Autodesk Fusion 360 part; units mm, degrees
note: some values were not read from the file. Set by a fixed rule: which sketch regions a step uses.
(part 3 of 3)
sketch "Sketch8" plane through (0, 0, 0) normal (0, 0, -1) x (1, 0, 0)
  line L0 (182.6113, -19.0647) -> (183.6113, -17.3326)
  line L1 (183.6113, -17.3326) -> (182.6113, -15.6006)
  line L2 (182.6113, -15.6006) -> (183.6113, -13.8685)
  line L3 (183.6113, -13.8685) -> (182.6113, -12.1365)
  line L4 (182.6113, -12.1365) -> (183.6113, -10.4044)
  line L5 (183.6113, -10.4044) -> (182.6113, -8.6724)
  line L6 (182.6113, -8.6724) -> (183.6113, -6.9403)
  line L7 (183.6113, -6.9403) -> (182.6113, -5.2083)
  line L8 (182.6113, -5.2083) -> (183.6113, -3.4762)
  line L9 (183.6113, -3.4762) -> (182.6113, -1.7442)
  line L10 (182.6113, -1.7442) -> (183.6113, -0.0121)
  line L11 (183.6113, -0.0121) -> (183.6113, 1.6298)
  line L12 (183.6113, 1.6298) -> (176, 1.6298)
  line L13 (176, 1.6298) -> (176, -7.1298)
  arc A0 (173.5, -11.4599) -> (176, -7.1298) centre (171, -7.1298) ccw
  line L14 (173.5, -11.4599) -> (170.6456, -13.1079)
  arc A1 (170.6456, -13.1079) -> (170.1456, -13.9739) centre (171.1456, -13.9739) ccw
  line L15 (170.1456, -13.9739) -> (170.1456, -15.2165)
  arc A2 (169.9665, -15.4154) -> (170.1456, -15.2165) centre (169.9456, -15.2165) ccw
  line L16 (169.9665, -15.4154) -> (167.3665, -15.6887)
  arc A3 (167.1456, -15.4898) -> (167.3665, -15.6887) centre (167.3456, -15.4898) ccw
  line L17 (167.1456, -15.4898) -> (167.1456, -15.4119)
  line L18 (167.1456, -15.4119) -> (151.6323, -17.0424)
  line L19 (151.6323, -17.0424) -> (151.6323, -17.1623)
  arc A4 (151.4532, -17.3612) -> (151.6323, -17.1623) centre (151.4323, -17.1623) ccw
  line L20 (151.4532, -17.3612) -> (148.8532, -17.6345)
  arc A5 (148.6323, -17.4356) -> (148.8532, -17.6345) centre (148.8323, -17.4356) ccw
  line L21 (148.6323, -17.4356) -> (148.6323, -15.55)
  arc A6 (148.6323, -15.55) -> (148.3823, -15.3) centre (148.3823, -15.55) ccw
  line L22 (148.3823, -15.3) -> (148.1323, -15.3)
  spline S0 degree 5 poles (148.1323, -15.3) (148.4158, -14.6516) (148.9812, -13.354) (149.8244, -11.4057) (150.9388, -8.8038) (152.3141, -5.5444) (153.6703, -2.2771) (155.0058, 0.9987) (156.3196, 4.2834) (157.6127, 7.5765) (158.8598, 10.8079) (159.8388, 13.3845) (160.5594, 15.3025) (161.0282, 16.559) (161.2489, 17.1526) knots 0 0 0 0 0 0 0.1 0.2 0.3 0.4 0.5 0.6 0.7 0.8 0.9 0.989467 0.989467 0.989467 0.989467 0.989467 0.989467
  arc A7 (161.7176, 17.4784) -> (161.2489, 17.1526) centre (161.7176, 16.9784) ccw
  line L23 (161.7176, 17.4784) -> (162.4215, 17.4784)
  arc A8 (162.9139, 17.0652) -> (162.4215, 17.4784) centre (162.4215, 16.9784) ccw
  line L24 (162.9139, 17.0652) -> (165.3864, 3.043)
  arc A9 (165.3864, 3.043) -> (165.8788, 2.6298) centre (165.8788, 3.1298) ccw
  line L25 (165.8788, 2.6298) -> (184.9592, 2.6298)
  arc A10 (185.4592, 2.1298) -> (184.9592, 2.6298) centre (184.9592, 2.1298) ccw
  line L26 (185.4592, 2.1298) -> (185.4592, -0.0467)
  line L27 (185.4592, -0.0467) -> (186.4393, -1.7442)
  line L28 (186.4393, -1.7442) -> (185.4393, -3.4762)
  line L29 (185.4393, -3.4762) -> (186.4393, -5.2083)
  line L30 (186.4393, -5.2083) -> (185.4393, -6.9403)
  line L31 (185.4393, -6.9403) -> (186.4393, -8.6724)
  line L32 (186.4393, -8.6724) -> (185.4393, -10.4044)
  line L33 (185.4393, -10.4044) -> (186.4393, -12.1365)
  line L34 (186.4393, -12.1365) -> (185.4393, -13.8685)
  line L35 (185.4393, -13.8685) -> (186.4393, -15.6006)
  line L36 (186.4393, -15.6006) -> (185.4393, -17.3326)
  line L37 (185.4393, -17.3326) -> (186.4393, -19.0647)
  line L38 (186.4393, -19.0647) -> (185.4393, -20.7967)
  line L39 (185.4393, -20.7967) -> (189.0932, -28.2505)
  arc A11 (189.0932, -28.2505) -> (190.889, -29.3702) centre (190.889, -27.3702) ccw
  line L40 (190.889, -29.3702) -> (197.156, -29.3702)
  arc A12 (197.156, -29.3702) -> (202.156, -24.3702) centre (197.156, -24.3702) ccw
  line L41 (202.156, -24.3702) -> (202.156, 8.9998)
  line L42 (202.156, 8.9998) -> (186.578, 8.932)
  arc A13 (186.578, 8.932) -> (186.0802, 8.4298) centre (186.5802, 8.432) ccw
  line L43 (186.0802, 8.4298) -> (186.0859, 7.132)
  arc A14 (185.5859, 6.6298) -> (186.0859, 7.132) centre (185.5859, 7.1298) ccw
  line L44 (185.5859, 6.6298) -> (178.088, 6.6298)
  arc A15 (177.588, 7.1298) -> (178.088, 6.6298) centre (178.088, 7.1298) ccw
  line L45 (177.588, 7.1298) -> (177.588, 23.1298)
  arc A16 (178.088, 23.6298) -> (177.588, 23.1298) centre (178.088, 23.1298) ccw
  line L46 (178.088, 23.6298) -> (182.1978, 23.6298)
  arc A17 (182.6828, 23.2512) -> (182.1978, 23.6298) centre (182.1978, 23.1298) ccw
  line L47 (182.6828, 23.2512) -> (186.1089, 9.5607)
  arc A18 (186.1089, 9.5607) -> (186.5961, 9.1821) centre (186.5939, 9.6821) ccw
  line L48 (186.5961, 9.1821) -> (202.2039, 9.25)
  line L49 (202.2039, 9.25) -> (202.169, 22.6429)
  arc A19 (202.169, 22.6429) -> (197.169, 27.6298) centre (197.169, 22.6298) ccw
  line L50 (197.169, 27.6298) -> (116.6624, 27.6298)
  arc A20 (116.6624, 27.6298) -> (112.7407, 25.7315) centre (116.6624, 22.6298) ccw
  arc A21 (80.6073, 9.9709) -> (112.7407, 25.7315) centre (80.1774, 51.4853) ccw
  line L51 (80.6073, 9.9709) -> (11.9433, 12.5645)
  arc A22 (11.9433, 12.5645) -> (11.704, -12.452) centre (11.002, 0.0641) ccw
  line L52 (11.704, -12.452) -> (89.3732, -10.2649)
  arc A23 (113.1229, -26.2409) -> (89.3732, -10.2649) centre (89.45, -35.7917) ccw
  arc A24 (113.1229, -26.2409) -> (117.7597, -29.3702) centre (117.7597, -24.3702) ccw
  line L53 (117.7597, -29.3702) -> (142.6323, -29.3702)
  line L54 (142.6323, -29.3702) -> (142.6323, -24.3589)
  line L55 (142.6323, -24.3589) -> (142.1438, -24.3589)
  line L56 (142.1438, -24.3589) -> (122.6074, -23.9078)
  arc A25 (122.1189, -23.408) -> (122.6074, -23.9078) centre (122.6189, -23.408) ccw
  line L57 (122.1189, -23.408) -> (122.1189, -20.1187)
  arc A26 (122.3398, -19.9198) -> (122.1189, -20.1187) centre (122.3189, -20.1187) ccw
  line L58 (122.3398, -19.9198) -> (125.0294, -20.2025)
  arc A27 (125.1189, -20.3019) -> (125.0294, -20.2025) centre (125.0189, -20.3019) ccw
  line L59 (125.1189, -20.3019) -> (125.1189, -20.3318)
  arc A28 (125.1189, -20.3318) -> (125.298, -20.5307) centre (125.3189, -20.3318) ccw
  line L60 (125.298, -20.5307) -> (140.4114, -22.1192)
  arc A29 (140.4114, -22.1192) -> (140.6323, -21.9203) centre (140.4323, -21.9203) ccw
  line L61 (140.6323, -21.9203) -> (140.6323, -21.8424)
  line L62 (140.6323, -21.8424) -> (143.4532, -22.1389)
  arc A30 (143.6323, -22.3378) -> (143.4532, -22.1389) centre (143.4323, -22.3378) ccw
  line L63 (143.6323, -22.3378) -> (143.6323, -33.3702)
  arc A31 (143.1323, -33.8702) -> (143.6323, -33.3702) centre (143.1323, -33.3702) ccw
  line L64 (143.1323, -33.8702) -> (141.6323, -33.8702)
  arc A32 (141.6323, -33.8702) -> (141.1323, -34.3702) centre (141.6323, -34.3702) ccw
  line L65 (141.1323, -34.3702) -> (141.1323, -38.0378)
  arc A33 (141.1323, -38.0378) -> (141.7774, -38.5162) centre (141.6323, -38.0378) ccw
  arc A34 (150.4871, -38.5162) -> (141.7774, -38.5162) centre (146.1323, -52.8702) ccw
  arc A35 (150.4871, -38.5162) -> (151.1323, -38.0378) centre (150.6323, -38.0378) ccw
  line L66 (151.1323, -38.0378) -> (151.1323, -34.3702)
  arc A36 (151.1323, -34.3702) -> (150.6323, -33.8702) centre (150.6323, -34.3702) ccw
  line L67 (150.6323, -33.8702) -> (149.1323, -33.8702)
  arc A37 (148.6323, -33.3702) -> (149.1323, -33.8702) centre (149.1323, -33.3702) ccw
  line L68 (148.6323, -33.3702) -> (148.6323, -22.3378)
  arc A38 (148.8114, -22.1389) -> (148.6323, -22.3378) centre (148.8323, -22.3378) ccw
  line L69 (148.8114, -22.1389) -> (151.4114, -21.8656)
  arc A39 (151.6323, -22.0645) -> (151.4114, -21.8656) centre (151.4323, -22.0645) ccw
  line L70 (151.6323, -22.0645) -> (151.6323, -22.1424)
  line L71 (151.6323, -22.1424) -> (167.1456, -20.5119)
  line L72 (167.1456, -20.5119) -> (167.1456, -20.392)
  arc A40 (167.3247, -20.1931) -> (167.1456, -20.392) centre (167.3456, -20.392) ccw
  line L73 (167.3247, -20.1931) -> (169.9247, -19.9198)
  arc A41 (170.1456, -20.1187) -> (169.9247, -19.9198) centre (169.9456, -20.1187) ccw
  line L74 (170.1456, -20.1187) -> (170.1456, -23.408)
  arc A42 (169.6572, -23.9078) -> (170.1456, -23.408) centre (169.6456, -23.408) ccw
  line L75 (169.6572, -23.9078) -> (149.6323, -24.3702)
  line L76 (149.6323, -24.3702) -> (149.6323, -29.3702)
  line L77 (149.6323, -29.3702) -> (178.1615, -29.3702)
  arc A43 (178.1615, -29.3702) -> (179.9574, -28.2505) centre (178.1615, -27.3702) ccw
  line L78 (179.9574, -28.2505) -> (183.6113, -20.7967)
  line L79 (183.6113, -20.7967) -> (182.6113, -19.0647)
  arc A44 (122.93, 6.6298) -> (123.4224, 7.043) centre (122.93, 7.1298) ccw
  line L80 (122.93, 6.6298) -> (121.7059, 6.6298)
  arc A45 (121.2059, 7.1298) -> (121.7059, 6.6298) centre (121.7059, 7.1298) ccw
  line L81 (121.2059, 7.1298) -> (121.2059, 23.1298)
  arc A46 (121.7059, 23.6298) -> (121.2059, 23.1298) centre (121.7059, 23.1298) ccw
  line L82 (121.7059, 23.6298) -> (176.588, 23.6298)
  arc A47 (177.088, 23.1298) -> (176.588, 23.6298) centre (176.588, 23.1298) ccw
  line L83 (177.088, 23.1298) -> (177.088, 7.1298)
  arc A48 (176.588, 6.6298) -> (177.088, 7.1298) centre (176.588, 7.1298) ccw
  line L84 (176.588, 6.6298) -> (169.2352, 6.6298)
  arc A49 (168.7428, 7.043) -> (169.2352, 6.6298) centre (169.2352, 7.1298) ccw
  line L85 (168.7428, 7.043) -> (166.1554, 21.7167)
  arc A50 (166.1554, 21.7167) -> (165.663, 22.1298) centre (165.663, 21.6298) ccw
  line L86 (165.663, 22.1298) -> (126.5021, 22.1298)
  arc A51 (126.5021, 22.1298) -> (126.0097, 21.7167) centre (126.5021, 21.6298) ccw
  line L87 (126.0097, 21.7167) -> (123.4224, 7.043)
  arc A52 (115.1907, -6.5098) -> (117.6907, -10.8399) centre (120.1907, -6.5098) ccw
  line L88 (115.1907, -6.5098) -> (115.1907, 10.1247)
  arc A53 (115.2816, 11.0735) -> (115.1907, 10.1247) centre (120.1907, 10.1247) ccw
  line L89 (115.2816, 11.0735) -> (117.6301, 23.2247)
  arc A54 (118.121, 23.6298) -> (117.6301, 23.2247) centre (118.121, 23.1298) ccw
  line L90 (118.121, 23.6298) -> (120.2059, 23.6298)
  arc A55 (120.7059, 23.1298) -> (120.2059, 23.6298) centre (120.2059, 23.1298) ccw
  line L91 (120.7059, 23.1298) -> (120.7059, 7.1298)
  arc A56 (120.2059, 6.6298) -> (120.7059, 7.1298) centre (120.2059, 7.1298) ccw
  arc A57 (120.2059, 6.6298) -> (119.7059, 6.1298) centre (120.2059, 6.1298) ccw
  line L92 (119.7059, 6.1298) -> (119.7059, 3.1298)
  arc A58 (119.7059, 3.1298) -> (120.2059, 2.6298) centre (120.2059, 3.1298) ccw
  line L93 (120.2059, 2.6298) -> (126.2864, 2.6298)
  arc A59 (126.2864, 2.6298) -> (126.7788, 3.043) centre (126.2864, 3.1298) ccw
  line L94 (126.7788, 3.043) -> (129.2794, 17.2246)
  arc A60 (129.7718, 17.6378) -> (129.2794, 17.2246) centre (129.7718, 17.1378) ccw
  line L95 (129.7718, 17.6378) -> (130.7595, 17.6378)
  spline S1 degree 5 poles (144.1323, -15.3) (144.0034, -15.0117) (143.5692, -14.0387) (142.8329, -12.3782) (141.8006, -10.0246) (140.482, -6.9691) (139.0131, -3.4934) (137.5684, 0.0041) (136.1486, 3.5243) (134.7528, 7.0662) (133.3923, 10.5941) (132.3224, 13.424) (131.5314, 15.5453) (131.012, 16.9513) (130.7595, 17.6378) knots -0.94214 -0.94214 -0.94214 -0.94214 -0.94214 -0.94214 -0.9 -0.8 -0.7 -0.6 -0.5 -0.4 -0.3 -0.2 -0.1 -0.004792 -0.004792 -0.004792 -0.004792 -0.004792 -0.004792
  line L96 (144.1323, -15.3) -> (143.8823, -15.3)
  arc A61 (143.8823, -15.3) -> (143.6323, -15.55) centre (143.8823, -15.55) ccw
  line L97 (143.6323, -15.55) -> (143.6323, -17.4356)
  arc A62 (143.4114, -17.6345) -> (143.6323, -17.4356) centre (143.4323, -17.4356) ccw
  line L98 (143.4114, -17.6345) -> (140.8114, -17.3612)
  arc A63 (140.6323, -17.1623) -> (140.8114, -17.3612) centre (140.8323, -17.1623) ccw
  line L99 (140.6323, -17.1623) -> (140.6323, -17.2225)
  arc A64 (140.6323, -17.2225) -> (140.4532, -17.0236) centre (140.4323, -17.2225) ccw
  line L100 (140.4532, -17.0236) -> (125.3398, -15.4351)
  arc A65 (125.3398, -15.4351) -> (125.1189, -15.634) centre (125.3189, -15.634) ccw
  line L101 (125.1189, -15.634) -> (125.1189, -15.7119)
  line L102 (125.1189, -15.7119) -> (122.298, -15.4154)
  arc A66 (122.1189, -15.2165) -> (122.298, -15.4154) centre (122.3189, -15.2165) ccw
  line L103 (122.1189, -15.2165) -> (122.1189, -13.9739)
  arc A67 (122.1189, -13.9739) -> (121.6189, -13.1079) centre (121.1189, -13.9739) ccw
  line L104 (121.6189, -13.1079) -> (117.6907, -10.8399)
  arc A68 (143.4114, -19.6345) -> (143.6323, -19.4356) centre (143.4323, -19.4356) ccw
  line L105 (143.4114, -19.6345) -> (140.7218, -19.3518)
  arc A69 (140.6323, -19.2524) -> (140.7218, -19.3518) centre (140.7323, -19.2524) ccw
  line L106 (140.6323, -19.2524) -> (140.6323, -19.2225)
  arc A70 (140.6323, -19.2225) -> (140.4532, -19.0236) centre (140.4323, -19.2225) ccw
  line L107 (140.4532, -19.0236) -> (125.3398, -17.4351)
  arc A71 (125.3398, -17.4351) -> (125.1189, -17.634) centre (125.3189, -17.634) ccw
  line L108 (125.1189, -17.634) -> (125.1189, -17.7119)
  line L109 (125.1189, -17.7119) -> (122.298, -17.4154)
  arc A72 (122.1189, -17.2165) -> (122.298, -17.4154) centre (122.3189, -17.2165) ccw
  line L110 (122.1189, -17.2165) -> (122.1189, -16.1187)
  arc A73 (122.3398, -15.9198) -> (122.1189, -16.1187) centre (122.3189, -16.1187) ccw
  line L111 (122.3398, -15.9198) -> (125.1189, -16.2119)
  line L112 (125.1189, -16.2119) -> (125.1189, -16.3318)
  arc A74 (125.1189, -16.3318) -> (125.298, -16.5307) centre (125.3189, -16.3318) ccw
  line L113 (125.298, -16.5307) -> (140.4114, -18.1192)
  arc A75 (140.4114, -18.1192) -> (140.6323, -17.9203) centre (140.4323, -17.9203) ccw
  line L114 (140.6323, -17.9203) -> (140.6323, -17.8424)
  line L115 (140.6323, -17.8424) -> (143.4532, -18.1389)
  arc A76 (143.6323, -18.3378) -> (143.4532, -18.1389) centre (143.4323, -18.3378) ccw
  line L116 (143.6323, -18.3378) -> (143.6323, -19.4356)
  spline S2 degree 5 poles (131.6523, 17.4499) (131.871, 16.8829) (132.3693, 15.5934) (133.1481, 13.5859) (134.2095, 10.8681) (135.5564, 7.4521) (136.9701, 3.9054) (138.3903, 0.385) (139.8173, -3.108) (141.2507, -6.5745) (142.5604, -9.7063) (143.5856, -12.1354) (144.3238, -13.8732) (144.7729, -14.9268) (144.9323, -15.3) knots -0.978339 -0.978339 -0.978339 -0.978339 -0.978339 -0.978339 -0.9 -0.8 -0.7 -0.6 -0.5 -0.4 -0.3 -0.2 -0.1 -0.045074 -0.045074 -0.045074 -0.045074 -0.045074 -0.045074
  arc A77 (132.1188, 18.1298) -> (131.6523, 17.4499) centre (132.1188, 17.6298) ccw
  line L117 (132.1188, 18.1298) -> (160.1605, 18.1298)
  arc A78 (160.6285, 17.4538) -> (160.1605, 18.1298) centre (160.1605, 17.6298) ccw
  line L118 (160.6285, 17.4538) -> (159.9652, 15.6911)
  spline S3 degree 5 poles (150.5222, -8.0328) (150.5836, -7.8891) (150.9212, -7.0983) (151.5369, -5.6459) (152.4351, -3.5002) (153.6231, -0.6091) (155.0461, 2.9325) (156.4844, 6.5848) (157.7568, 9.8732) (158.7459, 12.4635) (159.4459, 14.3123) (159.8529, 15.3927) (159.9652, 15.6911) knots -0.722257 -0.722257 -0.722257 -0.722257 -0.722257 -0.722257 -0.7 -0.6 -0.5 -0.4 -0.3 -0.2 -0.1 -0.061951 -0.061951 -0.061951 -0.061951 -0.061951 -0.061951
  spline S4 degree 3 poles (147.3323, -15.3) (147.3606, -15.2315) (147.3889, -15.163) (147.4174, -15.0945) (147.7999, -14.1733) (148.2003, -13.2596) (148.603, -12.3469) (149.0343, -11.3694) (149.4682, -10.3932) (149.9035, -9.4176) (150.1094, -8.9559) (150.3157, -8.4943) (150.5222, -8.0328) knots 80.396364 80.396364 80.396364 80.396364 80.841267 80.841267 80.841267 86.826165 86.826165 86.826165 93.23622 93.23622 93.23622 96.269727 96.269727 96.269727 96.269727
  line L119 (147.3323, -15.3) -> (144.9323, -15.3)
  line L120 (151.6323, -20.1424) -> (167.1456, -18.5119)
  line L121 (167.1456, -18.5119) -> (167.1456, -18.392)
  arc A79 (167.3247, -18.1931) -> (167.1456, -18.392) centre (167.3456, -18.392) ccw
  line L122 (167.3247, -18.1931) -> (169.9247, -17.9198)
  arc A80 (170.1456, -18.1187) -> (169.9247, -17.9198) centre (169.9456, -18.1187) ccw
  line L123 (170.1456, -18.1187) -> (170.1456, -19.2165)
  arc A81 (169.9665, -19.4154) -> (170.1456, -19.2165) centre (169.9456, -19.2165) ccw
  line L124 (169.9665, -19.4154) -> (167.3665, -19.6887)
  arc A82 (167.1456, -19.4898) -> (167.3665, -19.6887) centre (167.3456, -19.4898) ccw
  line L125 (167.1456, -19.4898) -> (167.1456, -19.4119)
  line L126 (167.1456, -19.4119) -> (151.6323, -21.0424)
  line L127 (151.6323, -21.0424) -> (151.6323, -21.1623)
  arc A83 (151.4532, -21.3612) -> (151.6323, -21.1623) centre (151.4323, -21.1623) ccw
  line L128 (151.4532, -21.3612) -> (148.8532, -21.6345)
  arc A84 (148.6323, -21.4356) -> (148.8532, -21.6345) centre (148.8323, -21.4356) ccw
  line L129 (148.6323, -21.4356) -> (148.6323, -20.3378)
  arc A85 (148.8114, -20.1389) -> (148.6323, -20.3378) centre (148.8323, -20.3378) ccw
  line L130 (148.8114, -20.1389) -> (151.4114, -19.8656)
  arc A86 (151.6323, -20.0645) -> (151.4114, -19.8656) centre (151.4323, -20.0645) ccw
  line L131 (151.6323, -20.0645) -> (151.6323, -20.1424)
  line L132 (151.6323, -18.1424) -> (167.1456, -16.5119)
  line L133 (167.1456, -16.5119) -> (167.1456, -16.392)
  arc A87 (167.3247, -16.1931) -> (167.1456, -16.392) centre (167.3456, -16.392) ccw
  line L134 (167.3247, -16.1931) -> (169.9247, -15.9198)
  arc A88 (170.1456, -16.1187) -> (169.9247, -15.9198) centre (169.9456, -16.1187) ccw
  line L135 (170.1456, -16.1187) -> (170.1456, -17.2165)
  arc A89 (169.9665, -17.4154) -> (170.1456, -17.2165) centre (169.9456, -17.2165) ccw
  line L136 (169.9665, -17.4154) -> (167.3665, -17.6887)
  arc A90 (167.1456, -17.4898) -> (167.3665, -17.6887) centre (167.3456, -17.4898) ccw
  line L137 (167.1456, -17.4898) -> (167.1456, -17.4119)
  line L138 (167.1456, -17.4119) -> (151.6323, -19.0424)
  line L139 (151.6323, -19.0424) -> (151.6323, -19.1623)
  arc A91 (151.4532, -19.3612) -> (151.6323, -19.1623) centre (151.4323, -19.1623) ccw
  line L140 (151.4532, -19.3612) -> (148.8532, -19.6345)
  arc A92 (148.6323, -19.4356) -> (148.8532, -19.6345) centre (148.8323, -19.4356) ccw
  line L141 (148.6323, -19.4356) -> (148.6323, -18.3378)
  arc A93 (148.8114, -18.1389) -> (148.6323, -18.3378) centre (148.8323, -18.3378) ccw
  line L142 (148.8114, -18.1389) -> (151.4114, -17.8656)
  arc A94 (151.6323, -18.0645) -> (151.4114, -17.8656) centre (151.4323, -18.0645) ccw
  line L143 (151.6323, -18.0645) -> (151.6323, -18.1424)
  circle A95 centre (11.002, 0.0641) radius 7.5
  arc A96 (143.4114, -21.6345) -> (143.6323, -21.4356) centre (143.4323, -21.4356) ccw
  line L144 (143.4114, -21.6345) -> (140.7218, -21.3518)
  arc A97 (140.6323, -21.2524) -> (140.7218, -21.3518) centre (140.7323, -21.2524) ccw
  line L145 (140.6323, -21.2524) -> (140.6323, -21.2225)
  arc A98 (140.6323, -21.2225) -> (140.4532, -21.0236) centre (140.4323, -21.2225) ccw
  line L146 (140.4532, -21.0236) -> (125.3398, -19.4351)
  arc A99 (125.3398, -19.4351) -> (125.1189, -19.634) centre (125.3189, -19.634) ccw
  line L147 (125.1189, -19.634) -> (125.1189, -19.7119)
  line L148 (125.1189, -19.7119) -> (122.298, -19.4154)
  arc A100 (122.1189, -19.2165) -> (122.298, -19.4154) centre (122.3189, -19.2165) ccw
  line L149 (122.1189, -19.2165) -> (122.1189, -18.1187)
  arc A101 (122.3398, -17.9198) -> (122.1189, -18.1187) centre (122.3189, -18.1187) ccw
  line L150 (122.3398, -17.9198) -> (125.1189, -18.2119)
  line L151 (125.1189, -18.2119) -> (125.1189, -18.3318)
  arc A102 (125.1189, -18.3318) -> (125.298, -18.5307) centre (125.3189, -18.3318) ccw
  line L152 (125.298, -18.5307) -> (140.4114, -20.1192)
  arc A103 (140.4114, -20.1192) -> (140.6323, -19.9203) centre (140.4323, -19.9203) ccw
  line L153 (140.6323, -19.9203) -> (140.6323, -19.8424)
  line L154 (140.6323, -19.8424) -> (143.4532, -20.1389)
  arc A104 (143.6323, -20.3378) -> (143.4532, -20.1389) centre (143.4323, -20.3378) ccw
  line L155 (143.6323, -20.3378) -> (143.6323, -21.4356)
  line L156 (21.1868, -7.183) -> (81.002, -5.4987)
  line L157 (21.2587, 7.2091) -> (81.002, 4.9525)
  line L158 (81.002, -5.4987) -> (81.002, 4.9525)
  arc A105 (21.1868, -7.183) -> (21.2587, 7.2091) centre (11.002, 0.0641) ccw
  dimension "d175" = 25
  dimension "d176" = 5
  dimension "d177" = 5
  dimension "d178" = 70
  constraint concentric A22 A105
  constraint parallel L52 L156
  constraint parallel L51 L157
  constraint vertical L158
  measures "d175" diameter of A105
  measures "d176" distance of L52 L156
  measures "d177" distance of L51 L157
  measures "d178" distance of A22.centre L158
extrude "Extrude7" cut sketch "Sketch8" against normal blind 1 contours L156 L157 L158 A105
fillet "Fillet1" radius 1 8 edges at (51.0944, 6.3408, 1) (81.002, 0.2731, 1) (51.1303, -6.0808, 1) (23.5018, -0.0016, 1) (51.1303, -6.0808, 6) (23.5018, -0.0016, 6) (51.0944, 6.3408, 6) (81.002, 0.2731, 6)
equation "t = 1.5 mm"
equation "th = 4 mm"
equation "d19 = th"
equation "d21 = t"
equation "d22 = ss"
equation "ss = 0.5 mm"
equation "d24 = h"
equation "d25 = h"
equation "h = 17 mm"
equation "d27 = h"
equation "d28 = h"
equation "d29 = h"
equation "d30 = ss"
equation "d31 = mss"
equation "mss = 0.8 mm"
equation "d39 = ss"
equation "d40 = t"
equation "d41 = ss"
equation "d42 = t"
equation "d44 = ss"
equation "d46 = th"
equation "d50 = mss"
equation "d51 = ss"
equation "d52 = mss"
equation "d53 = ss"
equation "d57 = th"
equation "d61 = th"
equation "d62 = th"
equation "d85 = th"
equation "d112 = th"
equation "d116 = ( 1.828 / 2 ) * 1 mm"
equation "fil = 0.5 mm"
equation "d127 = fil"
equation "d129 = fil"
equation "d131 = fil"
